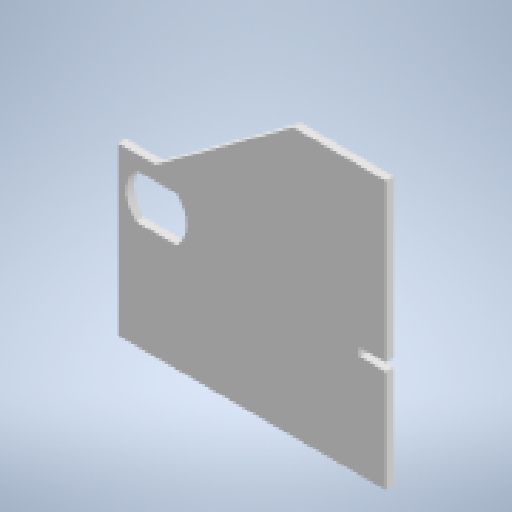
# Autodesk Inventor part: lr
Saved by Autodesk Inventor 2023.2 (Build 272271030, 271C)
## iProperties
Created: 2023-06-22
Part Number: lr
Material: Generic
Document SubType Name: Modeling
Designer: kao91
Density: 1 g/cm^3
Appearance: Default
Author: kao91
Autodesk Inventor part; units mm, degrees
ref_plane "YZ Plane" through (0, 0, 0) normal (1, 0, 0) x (0, 1, 0)
ref_plane "XZ Plane" through (0, 0, 0) normal (0, 1, 0) x (-1, 0, 0)
ref_plane "XY Plane" through (0, 0, 0) normal (0, 0, 1) x (1, 0, 0)
sketch "Sketch1" plane through (0, 0, 0) normal (0, 0, 1) x (1, 0, 0)
  line L0 (-54.0392, -39.25) -> (20.0037, -39.25)
  line L1 (10.0037, 0) -> (10.0037, 3)
  line L2 (10.0037, 0) -> (20.0037, 0)
  line L3 (10.0037, 3) -> (20.0037, 3)
  line L4 (10.0037, 0) -> (10.0037, 3)
  line L5 (10.0037, 0) -> (20.0037, 0)
  line L6 (20.0037, -39.25) -> (20.0037, 0)
  line L7 (20.0037, 3) -> (20.0037, 63)
  arc A0 (-54.0392, -39.25) -> (-53.6, -39.1535) centre (-67.7982, 24.405) ccw
  line L8 (20.0037, 63) -> (-15.3416, 63)
  line L9 (-54.0392, -39.25) -> (20.0037, -39.25) projected
  line L10 (20.0037, 3) -> (20.0037, 63) projected
  line L11 (20.0037, 63) -> (-15.3416, 63)
  line L12 (-81.9963, 3.828) -> (-81.9963, -39.1535)
  line L13 (-81.9963, -39.1535) -> (20.0037, -39.1535)
  line L14 (20.0037, -39.1535) -> (20.0037, 63)
  line L15 (-67.7982, 24.405) -> (-15.3416, 63)
  line L16 (-67.7982, 24.405) -> (-81.9963, 24.405)
  line L17 (-81.9963, 3.828) -> (-81.9963, 24.405)
  line L18 (-75.3539, 18.905) -> (-59.7432, 18.905) projected
  arc A1 (-75.3539, 18.905) -> (-75.3539, 1.905) centre (-67.4236, 10.405) ccw projected
  arc A2 (-59.7432, 1.905) -> (-59.7432, 18.905) centre (-67.6736, 10.405) ccw projected
  line L19 (-59.7432, 1.905) -> (-75.3539, 1.905) projected
  point P0 (0, 0)
  point P1 (10.0037, 1.5)
  point P2 (15.8221, 3)
  point P3 (31.7678, 19.4235)
  point P4 (31.6403, 19.4235)
  point P5 (31.6403, 19.4235)
  point P6 (20.0037, -39.1535)
  dimension "d2" = 35.3453
  dimension "d3" = 10
  dimension "d4" = 10
  dimension "d14" = 63.655
  dimension "d15" = 87.8019
  dimension "d16" = 0
  dimension "d17" = 0
  dimension "d18" = 3
  dimension "d19" = 60
  dimension "d20" = 102
  constraints: 32 end point, 5 perpendicular, 4 horizontal, 3 point on circle, 2 parallel, 2 point on line, 1 centre point, 1 coincident, 1 midpoint
  measures "d2" distance of L8.end L7.end
  measures "d3" distance between parallel lines of L1 L6
  measures "d4" distance between parallel lines of L1 L7
  measures "d14" distance from line of A0.centre L0
  measures "d15" distance from line of A0.centre L7
  measures "d16" distance between parallel lines of L9 L0
  measures "d17" distance between parallel lines of L10 L7
  measures "d18" distance between parallel lines of L2 L3
  measures "d19" distance between parallel lines of L8 L3
  measures "d20" distance of L13.end L12.end
extrude "Extrusion1" add sketch "Sketch1" along normal blind 3 contours L13 L12 L17 L16 L15 L8 L7 L3 L1 L2 L6 | L18 A2 L19 A1
body "Solid1"
